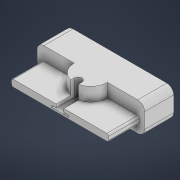
# Autodesk Inventor part: syringe_sledge_fitter
Saved by Autodesk Inventor 2022 (Build 260153000, 153)
## iProperties
Created: 2023-04-24
Part Number: syringe_sledge_fitter
Material: Generic
Document SubType Name: Modeling
Designer: Jakob Saugbjerg
Density: 1 g/cm^3
Appearance: Default
Author: Jakob Saugbjerg
Autodesk Inventor part; units mm, degrees
ref_plane "YZ Plane" through (0, 0, 0) normal (1, 0, 0) x (0, 1, 0)
ref_plane "XZ Plane" through (0, 0, 0) normal (0, 1, 0) x (-1, 0, 0)
ref_plane "XY Plane" through (0, 0, 0) normal (0, 0, 1) x (1, 0, 0)
sketch "Sketch1" plane through (0, 0, 0) normal (0, 0, 1) x (1, 0, 0)
  line L0 (0, 0) -> (63, 0)
  line L1 (63, 0) -> (63, 17)
  line L2 (63, 17) -> (0, 17)
  line L3 (0, 17) -> (0, 0)
  dimension "d0" = 63
  dimension "d1" = 17
  constraints: 8 end point, 2 parallel, 1 horizontal, 1 perpendicular
  measures "d0" distance of L2.end L1.end
  measures "d1" distance of L1.end L0.end
extrude "Extrusion1" add sketch "Sketch1" along normal blind 35
sketch "Sketch10" plane through (0, 0, 0) normal (0, 0, -1) x (-1, 0, 0)
  line L0 (-19.7584, 8.7843) -> (-18.2714, 8.7843)
  line L1 (-18.2714, 8.7843) -> (-18.2714, 8.4731)
  line L2 (-18.2714, 8.4731) -> (-18.8247, 8.4731)
  line L3 (-18.8247, 8.4731) -> (-18.8247, 6.4304)
  line L4 (-18.8247, 6.4304) -> (-18.2714, 6.4304)
  line L5 (-18.2714, 6.4304) -> (-18.2714, 6.1512)
  spline S0 degree 2 poles (-18.2714, 6.1512) (-18.5851, 6.1512) (-18.8815, 5.9734) (-18.9013, 5.7264) knots 0 0 0 1 2 2 2
  line L6 (-18.9013, 5.7264) -> (-19.2174, 5.7264)
  line L7 (-19.2174, 5.7264) -> (-19.2174, 8.4731)
  line L8 (-19.2174, 8.4731) -> (-19.7584, 8.4731)
  line L9 (-19.7584, 8.4731) -> (-19.7584, 8.7843)
  line L10 (-24.2785, 8.7843) -> (-24.2785, 7.4603)
  spline S1 degree 2 poles (-24.2785, 7.4603) (-24.2785, 7.3023) (-24.2538, 7.033) (-24.2143, 6.9589) knots 0 0 0 1 2 2 2
  spline S2 degree 2 poles (-24.2143, 6.9589) (-24.1748, 6.8774) (-24.0241, 6.7984) (-23.8932, 6.7984) knots 0 0 0 1 2 2 2
  spline S3 degree 2 poles (-23.8932, 6.7984) (-23.7746, 6.7984) (-23.5029, 6.9441) (-23.3597, 7.0824) knots 0 0 0 1 2 2 2
  spline S4 degree 2 poles (-23.3597, 7.0824) (-23.3621, 7.117) (-23.3671, 7.2133) (-23.3671, 7.2776) knots 0 0 0 1 2 2 2
  line L11 (-23.3671, 7.2776) -> (-23.3671, 8.7843)
  line L12 (-23.3671, 8.7843) -> (-22.9817, 8.7843)
  line L13 (-22.9817, 8.7843) -> (-22.9817, 7.4603)
  spline S5 degree 2 poles (-22.9817, 7.4603) (-22.9817, 7.3023) (-22.957, 7.033) (-22.9175, 6.9589) knots 0 0 0 1 2 2 2
  spline S6 degree 2 poles (-22.9175, 6.9589) (-22.878, 6.8774) (-22.7273, 6.7984) (-22.5964, 6.7984) knots 0 0 0 1 2 2 2
  spline S7 degree 2 poles (-22.5964, 6.7984) (-22.4729, 6.7984) (-22.1987, 6.954) (-22.0703, 7.075) knots 0 0 0 1 2 2 2
  line L14 (-22.0703, 7.075) -> (-22.0703, 8.7843)
  line L15 (-22.0703, 8.7843) -> (-21.685, 8.7843)
  line L16 (-21.685, 8.7843) -> (-21.685, 6.497)
  line L17 (-21.685, 6.497) -> (-22.0703, 6.497)
  line L18 (-22.0703, 6.497) -> (-22.0703, 6.749)
  spline S8 degree 2 poles (-22.0703, 6.749) (-22.221, 6.5983) (-22.5174, 6.4328) (-22.6952, 6.4328) knots 0 0 0 1 2 2 2
  spline S9 degree 2 poles (-22.6952, 6.4328) (-22.8978, 6.4328) (-23.2114, 6.6181) (-23.293, 6.828) knots 0 0 0 1 2 2 2
  spline S10 degree 2 poles (-23.293, 6.828) (-23.4683, 6.6329) (-23.7993, 6.4328) (-23.992, 6.4328) knots 0 0 0 1 2 2 2
  spline S11 degree 2 poles (-23.992, 6.4328) (-24.1402, 6.4328) (-24.3822, 6.5242) (-24.4712, 6.628) knots 0 0 0 1 2 2 2
  spline S12 degree 2 poles (-24.4712, 6.628) (-24.5625, 6.7317) (-24.6638, 7.0429) (-24.6638, 7.2776) knots 0 0 0 1 2 2 2
  line L19 (-24.6638, 7.2776) -> (-24.6638, 8.7843)
  line L20 (-24.6638, 8.7843) -> (-24.2785, 8.7843)
  line L21 (-27.0005, 8.7843) -> (-25.2344, 8.7843)
  line L22 (-25.2344, 8.7843) -> (-25.2344, 5.7363)
  line L23 (-25.2344, 5.7363) -> (-25.6395, 5.7363)
  line L24 (-25.6395, 5.7363) -> (-25.6395, 8.4237)
  line L25 (-25.6395, 8.4237) -> (-27.0005, 8.4237)
  line L26 (-27.0005, 8.4237) -> (-27.0005, 8.7843)
  spline S13 degree 2 poles (-29.2161, 8.8386) (-28.9863, 8.8386) (-28.5887, 8.7151) (-28.4578, 8.646) knots 0 0 0 1 2 2 2
  line L27 (-28.4578, 8.646) -> (-28.4578, 8.2137)
  line L28 (-28.4578, 8.2137) -> (-28.4775, 8.2137)
  spline S14 degree 2 poles (-28.4775, 8.2137) (-28.5269, 8.2532) (-28.6603, 8.3471) (-28.7715, 8.399) knots 0 0 0 1 2 2 2
  spline S15 degree 2 poles (-28.7715, 8.399) (-28.8678, 8.4459) (-29.1049, 8.515) (-29.2309, 8.515) knots 0 0 0 1 2 2 2
  spline S16 degree 2 poles (-29.2309, 8.515) (-29.3223, 8.515) (-29.5322, 8.4731) (-29.5816, 8.4385) knots 0 0 0 1 2 2 2
  spline S17 degree 2 poles (-29.5816, 8.4385) (-29.6533, 8.3915) (-29.7175, 8.2853) (-29.7175, 8.1767) knots 0 0 0 1 2 2 2
  spline S18 degree 2 poles (-29.7175, 8.1767) (-29.7175, 8.0408) (-29.5693, 7.9) (-29.3791, 7.8531) knots 0 0 0 1 2 2 2
  spline S19 degree 2 poles (-29.3791, 7.8531) (-29.305, 7.8358) (-29.0679, 7.7864) (-28.9666, 7.7592) knots 0 0 0 1 2 2 2
  spline S20 degree 2 poles (-28.9666, 7.7592) (-28.7048, 7.6826) (-28.4676, 7.3665) (-28.4676, 7.1417) knots 0 0 0 1 2 2 2
  spline S21 degree 2 poles (-28.4676, 7.1417) (-28.4676, 6.8305) (-28.9345, 6.4427) (-29.3198, 6.4427) knots 0 0 0 1 2 2 2
  spline S22 degree 2 poles (-29.3198, 6.4427) (-29.51, 6.4427) (-29.8953, 6.5366) (-30.0262, 6.6082) knots 0 0 0 1 2 2 2
  line L29 (-30.0262, 6.6082) -> (-30.0262, 7.0207)
  line L30 (-30.0262, 7.0207) -> (-30.0065, 7.0207)
  spline S23 degree 2 poles (-30.0065, 7.0207) (-29.8583, 6.9021) (-29.4976, 6.7663) (-29.3124, 6.7663) knots 0 0 0 1 2 2 2
  spline S24 degree 2 poles (-29.3124, 6.7663) (-29.1222, 6.7663) (-28.8604, 6.9268) (-28.8604, 7.0874) knots 0 0 0 1 2 2 2
  spline S25 degree 2 poles (-28.8604, 7.0874) (-28.8604, 7.2331) (-29.016, 7.3739) (-29.1889, 7.4184) knots 0 0 0 1 2 2 2
  spline S26 degree 2 poles (-29.1889, 7.4184) (-29.2729, 7.4406) (-29.4853, 7.485) (-29.6014, 7.5122) knots 0 0 0 1 2 2 2
  spline S27 degree 2 poles (-29.6014, 7.5122) (-29.8533, 7.5764) (-30.1102, 7.8704) (-30.1102, 8.1248) knots 0 0 0 1 2 2 2
  spline S28 degree 2 poles (-30.1102, 8.1248) (-30.1102, 8.273) (-29.9941, 8.5348) (-29.8805, 8.6311) knots 0 0 0 1 2 2 2
  spline S29 degree 2 poles (-29.8805, 8.6311) (-29.7595, 8.7324) (-29.4507, 8.8386) (-29.2161, 8.8386) knots 0 0 0 1 2 2 2
  line L31 (-32.2641, 6.497) -> (-31.034, 9.6266)
  line L32 (-31.034, 9.6266) -> (-30.6215, 9.6266)
  line L33 (-30.6215, 9.6266) -> (-31.0315, 8.6731)
  line L34 (-31.0315, 8.6731) -> (-30.2016, 6.497)
  line L35 (-30.2016, 6.497) -> (-30.6166, 6.497)
  line L36 (-30.6166, 6.497) -> (-31.2415, 8.1915)
  line L37 (-31.2415, 8.1915) -> (-31.8639, 6.497)
  line L38 (-31.8639, 6.497) -> (-32.2641, 6.497)
  line L39 (-33.7683, 6.9095) -> (-33.7485, 6.9095)
  spline S30 degree 2 poles (-33.7485, 6.9095) (-33.7041, 6.8972) (-33.6077, 6.8922) (-33.5411, 6.8922) knots 0 0 0 1 2 2 2
  spline S31 degree 2 poles (-33.5411, 6.8922) (-33.3854, 6.8922) (-33.0792, 7.0281) (-32.9408, 7.1615) knots 0 0 0 1 2 2 2
  line L40 (-32.9408, 7.1615) -> (-32.9408, 8.7843)
  line L41 (-32.9408, 8.7843) -> (-32.5555, 8.7843)
  line L42 (-32.5555, 8.7843) -> (-32.5555, 6.497)
  line L43 (-32.5555, 6.497) -> (-32.9408, 6.497)
  line L44 (-32.9408, 6.497) -> (-32.9408, 6.8379)
  spline S32 degree 2 poles (-32.9408, 6.8379) (-33.1508, 6.6502) (-33.4645, 6.497) (-33.6127, 6.497) knots 0 0 0 1 2 2 2
  spline S33 degree 2 poles (-33.6127, 6.497) (-33.672, 6.497) (-33.7312, 6.502) (-33.7683, 6.5094) knots 0 0 0 1 2 2 2
  line L45 (-33.7683, 6.5094) -> (-33.7683, 6.9095)
  line L46 (-34.4599, 8.7843) -> (-34.0746, 8.7843)
  line L47 (-34.0746, 8.7843) -> (-34.0746, 6.497)
  line L48 (-34.0746, 6.497) -> (-34.4599, 6.497)
  line L49 (-34.4599, 6.497) -> (-34.4599, 8.7843)
  line L50 (-34.4871, 6.1167) -> (-34.0499, 6.1167)
  line L51 (-34.0499, 6.1167) -> (-34.0499, 5.7165)
  line L52 (-34.0499, 5.7165) -> (-34.4871, 5.7165)
  line L53 (-34.4871, 5.7165) -> (-34.4871, 6.1167)
  line L54 (-36.8212, 8.7843) -> (-36.4359, 8.7843)
  line L55 (-36.4359, 8.7843) -> (-36.4359, 7.4801)
  spline S34 degree 2 poles (-36.4359, 7.4801) (-36.4359, 7.322) (-36.4063, 7.0503) (-36.3618, 6.9688) knots 0 0 0 1 2 2 2
  spline S35 degree 2 poles (-36.3618, 6.9688) (-36.3149, 6.8824) (-36.1469, 6.7984) (-36.0037, 6.7984) knots 0 0 0 1 2 2 2
  spline S36 degree 2 poles (-36.0037, 6.7984) (-35.8604, 6.7984) (-35.5566, 6.9515) (-35.4109, 7.075) knots 0 0 0 1 2 2 2
  line L56 (-35.4109, 7.075) -> (-35.4109, 8.7843)
  line L57 (-35.4109, 8.7843) -> (-35.0255, 8.7843)
  line L58 (-35.0255, 8.7843) -> (-35.0255, 6.497)
  line L59 (-35.0255, 6.497) -> (-35.4109, 6.497)
  line L60 (-35.4109, 6.497) -> (-35.4109, 6.7515)
  spline S37 degree 2 poles (-35.4109, 6.7515) (-35.5838, 6.5958) (-35.9172, 6.4328) (-36.1049, 6.4328) knots 0 0 0 1 2 2 2
  spline S38 degree 2 poles (-36.1049, 6.4328) (-36.4409, 6.4328) (-36.8212, 6.8774) (-36.8212, 7.2998) knots 0 0 0 1 2 2 2
  line L61 (-36.8212, 7.2998) -> (-36.8212, 8.7843)
  spline S39 degree 2 poles (-37.4437, 9.1498) (-37.4832, 9.1671) (-37.6339, 9.2215) (-37.7302, 9.2437) knots 0 0 0 1 2 2 2
  spline S40 degree 2 poles (-37.7302, 9.2437) (-37.8364, 9.2709) (-38.0167, 9.303) (-38.1229, 9.303) knots 0 0 0 1 2 2 2
  spline S41 degree 2 poles (-38.1229, 9.303) (-38.3008, 9.303) (-38.5478, 9.2091) (-38.6169, 9.1251) knots 0 0 0 1 2 2 2
  spline S42 degree 2 poles (-38.6169, 9.1251) (-38.6836, 9.0412) (-38.7355, 8.8213) (-38.7355, 8.6805) knots 0 0 0 1 2 2 2
  line L62 (-38.7355, 8.6805) -> (-38.7355, 8.4805)
  spline S43 degree 2 poles (-38.7355, 8.4805) (-38.5799, 8.6163) (-38.281, 8.7448) (-38.0562, 8.7448) knots 0 0 0 1 2 2 2
  spline S44 degree 2 poles (-38.0562, 8.7448) (-37.666, 8.7448) (-37.2041, 8.1643) (-37.2041, 7.6184) knots 0 0 0 1 2 2 2
  spline S45 degree 2 poles (-37.2041, 7.6184) (-37.2041, 7.3344) (-37.3646, 6.8947) (-37.498, 6.7391) knots 0 0 0 1 2 2 2
  spline S46 degree 2 poles (-37.498, 6.7391) (-37.6265, 6.5934) (-37.9797, 6.4328) (-38.1674, 6.4328) knots 0 0 0 1 2 2 2
  spline S47 degree 2 poles (-38.1674, 6.4328) (-38.3452, 6.4328) (-38.6046, 6.5168) (-38.7355, 6.5934) knots 0 0 0 1 2 2 2
  line L63 (-38.7355, 6.5934) -> (-38.7577, 6.497)
  line L64 (-38.7577, 6.497) -> (-39.1208, 6.497)
  line L65 (-39.1208, 6.497) -> (-39.1208, 8.5225)
  spline S48 degree 2 poles (-39.1208, 8.5225) (-39.1208, 9.1054) (-38.6145, 9.6488) (-38.0933, 9.6488) knots 0 0 0 1 2 2 2
  spline S49 degree 2 poles (-38.0933, 9.6488) (-37.9253, 9.6488) (-37.5746, 9.5944) (-37.4239, 9.55) knots 0 0 0 1 2 2 2
  line L66 (-37.4239, 9.55) -> (-37.4239, 9.1498)
  line L67 (-37.4239, 9.1498) -> (-37.4437, 9.1498)
  line L68 (-38.7355, 8.1643) -> (-38.7355, 6.9071)
  spline S50 degree 2 poles (-38.7355, 6.9071) (-38.5922, 6.8379) (-38.3502, 6.7786) (-38.2291, 6.7786) knots 0 0 0 1 2 2 2
  spline S51 degree 2 poles (-38.2291, 6.7786) (-37.9377, 6.7786) (-37.6018, 7.2084) (-37.6018, 7.611) knots 0 0 0 1 2 2 2
  spline S52 degree 2 poles (-37.6018, 7.611) (-37.6018, 7.9914) (-37.8562, 8.3891) (-38.1427, 8.3891) knots 0 0 0 1 2 2 2
  spline S53 degree 2 poles (-38.1427, 8.3891) (-38.2934, 8.3891) (-38.6095, 8.2705) (-38.7355, 8.1643) knots 0 0 0 1 2 2 2
  spline S54 degree 2 poles (-40.672, 8.8361) (-40.1237, 8.8361) (-39.521, 8.2211) (-39.521, 7.653) knots 0 0 0 1 2 2 2
  spline S55 degree 2 poles (-39.521, 7.653) (-39.521, 7.0948) (-40.1064, 6.4328) (-40.5781, 6.4328) knots 0 0 0 1 2 2 2
  spline S56 degree 2 poles (-40.5781, 6.4328) (-40.7906, 6.4328) (-41.1191, 6.5563) (-41.2401, 6.6872) knots 0 0 0 1 2 2 2
  spline S57 degree 2 poles (-41.2401, 6.6872) (-41.3636, 6.8181) (-41.4945, 7.1961) (-41.4945, 7.4702) knots 0 0 0 1 2 2 2
  line L69 (-41.4945, 7.4702) -> (-41.4945, 7.6802)
  line L70 (-41.4945, 7.6802) -> (-39.9112, 7.6802)
  spline S58 degree 2 poles (-39.9112, 7.6802) (-39.9112, 8.0779) (-40.3114, 8.5002) (-40.6671, 8.5002) knots 0 0 0 1 2 2 2
  spline S59 degree 2 poles (-40.6671, 8.5002) (-40.793, 8.5002) (-41.0376, 8.4434) (-41.1364, 8.399) knots 0 0 0 1 2 2 2
  spline S60 degree 2 poles (-41.1364, 8.399) (-41.2401, 8.3496) (-41.3834, 8.2631) (-41.4303, 8.2236) knots 0 0 0 1 2 2 2
  line L71 (-41.4303, 8.2236) -> (-41.4525, 8.2236)
  line L72 (-41.4525, 8.2236) -> (-41.4525, 8.6435)
  spline S61 degree 2 poles (-41.4525, 8.6435) (-41.3858, 8.6707) (-41.1833, 8.7497) (-41.1042, 8.7719) knots 0 0 0 1 2 2 2
  spline S62 degree 2 poles (-41.1042, 8.7719) (-40.9931, 8.804) (-40.8103, 8.8361) (-40.672, 8.8361) knots 0 0 0 1 2 2 2
  spline S63 degree 2 poles (-41.1191, 7.3862) (-41.1141, 7.2306) (-41.0499, 7.0034) (-40.9882, 6.9268) knots 0 0 0 1 2 2 2
  spline S64 degree 2 poles (-40.9882, 6.9268) (-40.9215, 6.8404) (-40.7115, 6.749) (-40.5559, 6.749) knots 0 0 0 1 2 2 2
  spline S65 degree 2 poles (-40.5559, 6.749) (-40.4028, 6.749) (-40.1879, 6.8404) (-40.099, 6.9293) knots 0 0 0 1 2 2 2
  spline S66 degree 2 poles (-40.099, 6.9293) (-40.0125, 7.0207) (-39.9236, 7.2405) (-39.9112, 7.3862) knots 0 0 0 1 2 2 2
  line L73 (-39.9112, 7.3862) -> (-41.1191, 7.3862)
  point P0 (0, 0)
  point P1 (-17.8095, 5.7165)
  dimension "d3" = 0
  constraints: 1 other
emboss "Emboss1" sketch "Sketch10" operation cut depth 1 direction (0, 0, 1)
sketch "Sketch15" plane through (0, 0, 35) normal (0, 0, 1) x (1, 0, 0)
  line L0 (0, 17) -> (0, 0) projected
  line L1 (0, 0) -> (0, 5)
  line L2 (63, 0) -> (63, 17) projected
  line L3 (0, 5) -> (63, 5)
  line L4 (63, 5) -> (63, 0)
  line L5 (63, 0) -> (0, 0)
  line L6 (0, 0) -> (0, 5)
  line L7 (63, 17) -> (0, 17) projected
  line L8 (63, 17) -> (0, 17)
  line L9 (0, 17) -> (0, 9)
  line L10 (0, 9) -> (63, 9)
  line L11 (63, 9) -> (63, 17)
  dimension "d67" = 5
  dimension "d68" = 8
  constraints: 18 end point, 4 parallel, 2 horizontal, 2 perpendicular, 2 point on line
  measures "d67" distance of L0.end L1.end
  measures "d68" distance of L9.end L8.end
extrude "Extrusion12" cut sketch "Sketch15" against normal blind 18 contours L7 L2 L10 L0 | L3 L2 L5 L0
sketch "Sketch16" plane through (0, 9, 35) normal (0, 1, 0) x (1, 0, 0)
  line L0 (63, 0) -> (0, 0) projected
  line L1 (31.5, 0) -> (31.5, 8.25)
  line L2 (31.5, 8.25) -> (31.5, 10.5)
  circle A0 centre (31.5, 10.5) radius 2.25
  line L3 (29.25, 10.5) -> (33.75, 10.5)
  line L4 (33.75, 10.5) -> (33.75, 0)
  line L5 (33.75, 0) -> (29.25, 0)
  line L6 (29.25, 0) -> (29.25, 10.5)
  point P0 (0, 35)
  point P1 (33.75, 10.5)
  dimension "d90" = 8.25
  dimension "d91" = 2.25
  constraints: 12 end point, 2 parallel, 2 point on circle, 2 point on line, 1 centre point, 1 coincident, 1 horizontal, 1 midpoint, 1 perpendicular, 1 vertical
  measures "d90" distance of L1.start L1.end
  measures "d91" distance of L1.end L2.end
extrude "Extrusion13" cut sketch "Sketch16" against normal blind 2
sketch "Sketch17" plane through (0, 7, 35) normal (0, 1, 0) x (1, 0, 0)
  arc A0 (33.75, 10.5) -> (29.25, 10.5) centre (31.5, 10.5) ccw projected
  circle A1 centre (31.5, 10.5) radius 2.25
  circle A2 centre (31.5, 10.5) radius 5
  line L0 (29.25, 0) -> (0, 0) projected
  line L1 (36.5, 10.5) -> (26.5, 10.5)
  line L2 (26.5, 10.5) -> (26.5, 0)
  line L3 (26.5, 0) -> (36.5, 0)
  line L4 (36.5, 0) -> (36.5, 10.5)
  point P0 (0, 35)
  dimension "d92" = 10
  dimension "d93" = 10
  constraints: 8 end point, 2 coincident, 2 parallel, 2 point on circle, 1 centre point, 1 horizontal, 1 horizontal alignment, 1 perpendicular, 1 point on line, 2 other
  measures "d92" diameter of A2
  measures "d93" distance of L3.end L2.end
extrude "Extrusion14" cut sketch "Sketch17" against normal blind 1
sketch "Sketch18" plane through (0, 0, 35) normal (0, 0, 1) x (1, 0, 0)
  line L0 (0, 5) -> (63, 5) projected
  line L1 (3.1, 9) -> (59.9, 9)
  line L2 (59.9, 9) -> (59.9, 5)
  line L3 (59.9, 5) -> (3.1, 5)
  line L4 (3.1, 5) -> (3.1, 9)
  line L5 (3.1, 9) -> (59.9, 5) construction
  line L6 (59.9, 9) -> (3.1, 5) construction
  line L7 (63, 9) -> (0, 9) projected
  line L8 (59.9, 5) -> (63, 5)
  line L9 (63, 5) -> (63, 9)
  line L10 (63, 9) -> (59.9, 9)
  line L11 (59.9, 9) -> (59.9, 5)
  line L12 (0, 17) -> (0, 0) projected
  line L13 (3.1, 5) -> (0, 5)
  line L14 (0, 5) -> (0, 9)
  line L15 (0, 9) -> (3.1, 9)
  line L16 (3.1, 9) -> (3.1, 5)
  point P0 (31.5, 7)
  point P1 (37.25, 7)
  point P2 (3.1, 5)
  dimension "d78" = 56.8
  constraints: 26 end point, 5 parallel, 3 horizontal, 3 point on line, 2 midpoint, 2 perpendicular, 1 vertical, 4 other
  measures "d78" distance of L2.end L3.end
extrude "Extrusion15" cut sketch "Sketch18" against normal blind 18 contours L12 L7 L4 L0 | L2 L7 L9 L0
fillet "Fillet6" radius 1 4 edges at (3.1, 9, 26) (3.1, 5, 26) (59.9, 5, 26) (59.9, 9, 26)
fillet "Fillet7" radius 4 4 edges at (63, 17, 8.5) (63, 0, 8.5) (0, 0, 8.5) (0, 17, 8.5)
sketch "Sketch19" plane through (31.5, 9, 27.75) normal (0, 1, 0) x (1, 0, 0)
  line L0 (31.5, 10.75) -> (-31.5, 10.75) projected
  circle A0 centre (0, 10.75) radius 9.75
  arc A1 (2.25, 3.25) -> (-2.25, 3.25) centre (0, 3.25) ccw projected
  circle A2 centre (0, 3.25) radius 2.25
  line L1 (2.25, 3.25) -> (2.25, -7.25) projected
  line L2 (-2.25, -7.25) -> (-2.25, 3.25) projected
  line L3 (2.25, 3.25) -> (-2.25, 3.25)
  line L4 (-2.25, 3.25) -> (-2.25, 0.7968)
  line L5 (-2.25, 0.7968) -> (2.25, 0.7968)
  line L6 (2.25, 0.7968) -> (2.25, 3.25)
  point P0 (-31.5, 27.75)
  point P1 (27.4, 10.75)
  point P2 (-27.4, 10.75)
  point P3 (4.5, 0)
  point P4 (9.75, 10.75)
  point P5 (-9.75, 10.75)
  point P6 (-2.2493, 3.3077)
  point P7 (2.2493, 3.3077)
  point P8 (-2.25, 1.2632)
  point P9 (-2.2493, 3.3077)
  point P10 (2.2493, 3.3077)
  point P11 (2.25, 1.2632)
  point P12 (2.25, -1.2151)
  dimension "d84" = 19.5
  constraints: 8 end point, 2 centre point, 2 parallel, 1 coincident, 1 horizontal, 1 midpoint, 1 perpendicular, 1 point on line
  measures "d84" diameter of A0
extrude "Extrusion16" add sketch "Sketch19" along normal blind 8 contours A0 L1 A1 L2 L0 | L0 A0
body "Solid1"
